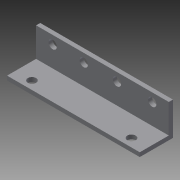
# Autodesk Inventor part: Connection to frame
Saved by Autodesk Inventor 2014 SP1 (Build 180222100, 222)
## iProperties
Created: 2014-01-16
Part Number: Connection to frame
Material: Generic
Document SubType Name: Modeling
Designer: JU BRIAN
Density: 1 g/cm^3
Appearance: Default
Author: JU BRIAN
Autodesk Inventor part; units mm, degrees
ref_plane "YZ Plane" through (0, 0, 0) normal (1, 0, 0) x (0, 1, 0)
ref_plane "XZ Plane" through (0, 0, 0) normal (0, 1, 0) x (-1, 0, 0)
ref_plane "XY Plane" through (0, 0, 0) normal (0, 0, 1) x (1, 0, 0)
sketch "Sketch1" plane through (0, 0, 0) normal (0, 1, 0) x (-1, 0, 0)
  line L0 (-13.6552, 6.526) -> (87.9448, 6.526)
  line L1 (87.9448, 6.526) -> (87.9448, -18.874)
  line L2 (87.9448, -18.874) -> (-13.6552, -18.874)
  line L3 (-13.6552, -18.874) -> (-13.6552, 6.526)
  dimension "d0" = 101.6
  dimension "d1" = 25.4
  constraints: 8 end point, 2 parallel, 1 horizontal, 1 perpendicular
  measures "d0" distance of L1.end L2.end
  measures "d1" distance of L0.end L1.end
extrude "Extrusion1" add sketch "Sketch1" along normal blind 3.175
sketch "Sketch2" plane through (0, 3.175, 0) normal (0, 1, 0) x (1, 0, 0)
  line L0 (-87.9448, 18.874) -> (13.6552, 18.874)
  line L1 (13.6552, 18.874) -> (13.6552, 15.699)
  line L2 (13.6552, 15.699) -> (-87.9448, 15.699)
  line L3 (-87.9448, 15.699) -> (-87.9448, 18.874)
  dimension "d4" = 101.6
  dimension "d5" = 3.175
  constraints: 8 end point, 2 parallel, 1 horizontal, 1 perpendicular
  measures "d4" distance of L1.end L2.end
  measures "d5" distance of L0.end L1.end
extrude "Extrusion2" add sketch "Sketch2" along normal blind 22.225
sketch "Sketch3" plane through (0, 3.175, 0) normal (0, 1, 0) x (1, 0, 0)
  line L0 (-87.9448, 15.699) -> (-87.9448, -6.526) projected
  line L1 (-87.9448, -6.526) -> (13.6552, -6.526) projected
  line L2 (13.6552, -6.526) -> (13.6552, 15.699) projected
  point P0 (-75.2448, -0.176)
  point P1 (0.9552, -0.176)
  dimension "d8" = 12.7
  dimension "d9" = 12.7
  dimension "d10" = 6.35
  constraints: 1 horizontal alignment
  measures "d8" distance from line of L2 point (0.955, -0.176)
  measures "d9" distance from line of L0 point (-75.245, -0.176)
  measures "d10" distance from line of L1 point (-75.245, -0.176)
hole "Hole1" at (-75.2448, 3.175, 0.176) at (0.9552, 3.175, 0.176) direction (0, -1, 0) diameter 6.35 end through all
sketch "Sketch4" plane through (-87.9448, 3.175, -15.699) normal (0, 0, 1) x (1, 0, 0)
  line L0 (0, 22.225) -> (101.6, 22.225) projected
  line L1 (101.6, 0) -> (101.6, 22.225) projected
  line L2 (0, 0) -> (0, 22.225) projected
  point P0 (12.7, 15.875)
  point P1 (88.9, 15.875)
  point P2 (61.9125, 15.875)
  point P3 (36.5125, 15.875)
  dimension "d18" = 6.35
  dimension "d26" = 39.6875
  dimension "d27" = 36.5125
  constraints: 1 horizontal alignment
  measures "d18" distance from line of L0 point (12.7, 15.875)
  measures "d26" distance from line of point (61.913, 15.875) L1
  measures "d27" distance from line of L2 point (36.513, 15.875)
hole "Hole2" at (-75.2448, 19.05, -15.699) at (0.9552, 19.05, -15.699) at (-51.4323, 19.05, -15.699) at (-26.0323, 19.05, -15.699) direction (0, 0, -1) diameter 6.35 end through all
body "Solid1"
